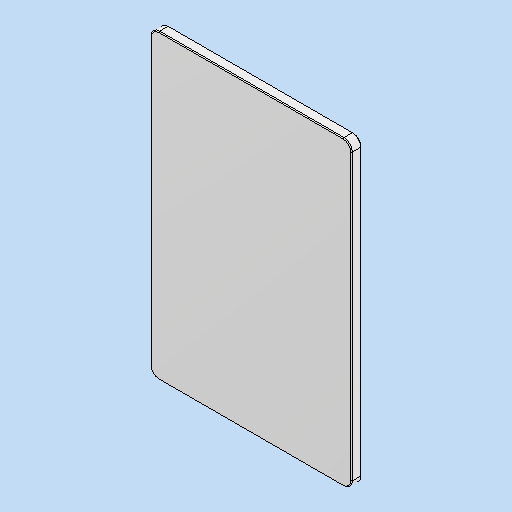
# Autodesk Inventor part: tc-bottom-tray
Saved by Autodesk Inventor 2025 (Build 290162000, 162)
## iProperties
Created: 2025-06-05
Part Number: tc-bottom-tray
Material: ABS Plastic
Document SubType Name: Modeling
Designer: queezz
Density: 1.06 g/cm^3
Appearance: Smooth - White
Author: queezz
Autodesk Inventor part; units mm, degrees
ref_plane "YZ Plane" through (0, 0, 0) normal (1, 0, 0) x (0, 1, 0)
ref_plane "XZ Plane" through (0, 0, 0) normal (0, 1, 0) x (-1, 0, 0)
ref_plane "XY Plane" through (0, 0, 0) normal (0, 0, 1) x (1, 0, 0)
sketch "Sketch1" plane through (0, 0, 0) normal (0, 0, 1) x (1, 0, 0)
  line L0 (-60, 90) -> (60, 90)
  line L1 (60, 90) -> (60, -90)
  line L2 (60, -90) -> (-60, -90)
  line L3 (-60, -90) -> (-60, 90)
  point P0 (0, 0)
  point P1 (60, 0)
  point P2 (0, 90)
  dimension "d0" = 120
  dimension "d1" = 180
  constraints: 8 end point, 2 midpoint, 2 parallel, 1 horizontal, 1 horizontal alignment, 1 perpendicular, 1 vertical alignment
  measures "d0" distance of L0.start L0.end
  measures "d1" distance of L0.end L1.end
extrude "Extrusion1" add sketch "Sketch1" along normal blind 6
fillet "Fillet1" radius 5 4 edges at (-60, 90, 3) (60, 90, 3) (60, -90, 3) (-60, -90, 3)
chamfer "Chamfer2" distance 0.5 angle 45 16 edges at (0, 90, 6) (-58.5355, 88.5355, 6) (-60, 0, 6) (-58.5355, -88.5355, 6) (0, -90, 6) (58.5355, -88.5355, 6) (60, 0, 6) (58.5355, 88.5355, 6) (0, 90, 0) (-58.5355, 88.5355, 0) (-60, 0, 0) (-58.5355, -88.5355, 0) (0, -90, 0) (58.5355, -88.5355, 0) (60, 0, 0) (58.5355, 88.5355, 0)
sketch "Sketch3" plane through (0, 0, 6) normal (0, 0, 1) x (1, 0, 0)
  line L0 (60, 75) -> (62, 75)
  line L1 (62, 75) -> (62, -75)
  line L2 (62, -75) -> (60, -75)
  line L3 (60, -75) -> (60, 75)
  line L4 (60, -85) -> (60, 85) projected
  point P0 (0, 0)
  point P1 (62, 0)
  point P2 (60, 0)
  dimension "d12" = 150
  dimension "d13" = 2
  constraints: 8 end point, 3 midpoint, 2 parallel, 1 horizontal, 1 horizontal alignment, 1 perpendicular
  measures "d12" distance of L0.end L1.end
  measures "d13" distance of L0.start L0.end
equation "\"d0\" = width"
equation "\"d1\" = hight"
equation "\"hight\" = 180"
equation "\"width\" = 120"
body "Solid1"
